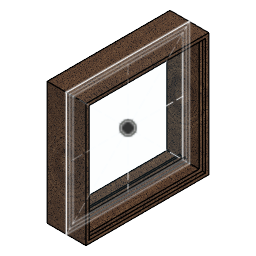
cutie (Autodesk Fusion 360 design; units mm, degrees)
part number: 2026-06-01-17-19-54-143
Autodesk Fusion 360 part; units mm, degrees
sketch "Sketch1" plane through (0, 0, 0) normal (1, 0, 0) x (0, 1, 0)
  line L0 (90, -90) -> (90, 90)
  line L1 (-95, 95) -> (95, -95) construction
  line L2 (95, 95) -> (-95, 95)
  line L3 (85, 85) -> (-85, 85)
  line L4 (-85, -85) -> (85, -85)
  line L5 (85, -85) -> (85, 85)
  line L6 (-95, 95) -> (-95, -95)
  line L7 (0, 85) -> (0, -85) construction
  line L8 (-85, 85) -> (-85, -85)
  line L9 (95, 95) -> (-95, -95) construction
  line L10 (95, -95) -> (95, 95)
  line L11 (90, 90) -> (-90, 90)
  line L12 (-90, -90) -> (90, -90)
  line L13 (-85, 0) -> (85, 0) construction
  line L14 (-95, -95) -> (95, -95)
  line L15 (-90, 90) -> (-90, -90)
  dimension "d3" = -5
  dimension "d4" = -5
  dimension "d5" = 190
  dimension "d6" = 190
  constraint horizontal L2
  constraint perpendicular L2 L6
  constraint parallel L2 L14
  constraint parallel L6 L10
  constraint coincident origin L9
  constraint coincident origin L1
  constraint midpoint L13.start L8
  constraint midpoint L13.end L5
  constraint midpoint L7.start L3
  constraint midpoint L7.end L4
  measures "d5" distance of L6.end L1.end
  measures "d6" distance of L1.start L6.end
extrude "Extrude4" add sketch "Sketch1" along normal mid plane 50 contours L0 L11 L12 L15
extrude "Extrude5" add sketch "Sketch1" along normal mid plane 60 contours L2 L6 L10 L14
sketch "Sketch2" plane through (0, 0, -85) normal (0, 0, 1) x (-1, 0, 0)
  line L0 (25, 85) -> (-25, 85)
  line L1 (-25, 85) -> (-25, -85)
  line L2 (-25, -85) -> (25, -85)
  line L3 (25, -85) -> (25, 85)
  line L4 (-2.525, 85) -> (2.525, 85)
  line L5 (2.525, 85) -> (2.525, -85)
  line L6 (2.525, -85) -> (-2.525, -85)
  line L7 (-2.525, -85) -> (-2.525, 85)
  line L8 (-2.525, 85) -> (2.525, -85) construction
  line L9 (2.525, 85) -> (-2.525, -85) construction
  line L10 (5.025, 87.5) -> (5.025, -87.5)
  line L11 (5.025, -87.5) -> (-5.025, -87.5)
  line L12 (-5.025, -87.5) -> (-5.025, 87.5)
  line L13 (-5.025, 87.5) -> (5.025, 87.5)
  dimension "d39" = -2.5
  dimension "d40" = 5.05
  constraint horizontal L4
  constraint perpendicular L4 L5
  constraint parallel L4 L6
  constraint parallel L5 L7
  constraint coincident L8 origin
  constraint coincident L9 origin
  constraint coincident L0 L4.start
  measures "d40" distance of L5 L7
extrude "Extrude6" add sketch "Sketch2" along normal blind 5 contours L0 L2 L5 L10 | L0 L2 L7 L12
sketch "Sketch3" plane through (0, 0, 85) normal (0, 0, -1) x (1, 0, 0)
  line L0 (-25, -85) -> (25, -85)
  line L1 (25, -85) -> (25, 85)
  line L2 (25, 85) -> (-25, 85)
  line L3 (-25, 85) -> (-25, -85)
  line L4 (-2.5, 85) -> (2.5, 85)
  line L5 (2.5, 85) -> (2.5, -85)
  line L6 (2.5, -85) -> (-2.5, -85)
  line L7 (-2.5, -85) -> (-2.5, 85)
  line L8 (-2.5, 85) -> (2.5, -85) construction
  line L9 (2.5, 85) -> (-2.5, -85) construction
  line L10 (5, 87.5) -> (5, -87.5)
  line L11 (5, -87.5) -> (-5, -87.5)
  line L12 (-5, -87.5) -> (-5, 87.5)
  line L13 (-5, 87.5) -> (5, 87.5)
  dimension "d43" = 5
  dimension "d44" = -2.5
  constraint horizontal L4
  constraint perpendicular L4 L5
  constraint parallel L4 L6
  constraint parallel L5 L7
  constraint coincident L8 origin
  constraint coincident L9 origin
  measures "d43" distance of L5.end L6.end
extrude "Extrude7" add sketch "Sketch3" along normal blind 5 contours L0 L2 L7 L12 | L0 L2 L5 L10
equation "d6 = d5"
named bodies: "Cutie mijloc"
